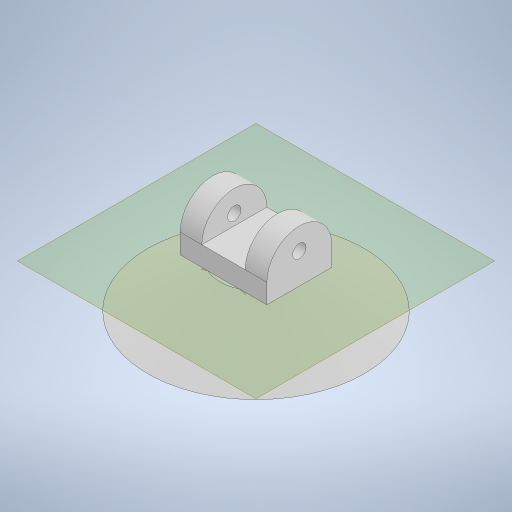
# Autodesk Inventor part: Деталь5
Saved by Autodesk Inventor 2023.1 (Build 271208000, 208)
## iProperties
Created: 2024-12-24
Part Number: Деталь5
Material: Типовые
Document SubType Name: Modeling
Designer: DELL
Density: 1 g/cm^3
Appearance: По умолчанию
Author: DELL
Autodesk Inventor part; units mm, degrees
ref_plane "YZ Plane" through (0, 0, 0) normal (1, 0, 0) x (0, 1, 0)
ref_plane "XZ Plane" through (0, 0, 0) normal (0, 1, 0) x (-1, 0, 0)
ref_plane "XY Plane" through (0, 0, 0) normal (0, 0, 1) x (1, 0, 0)
sketch "Эскиз2" plane through (0, 0, 0) normal (0, 0, 1) x (1, 0, 0)
  line L0 (0, 0) -> (25, 0)
  line L1 (0, 0) -> (0, 15)
  line L2 (0, 15) -> (25, 0)
  line L3 (0, -3) -> (0, 18) projected
  dimension "d0" = 25
  dimension "d1" = 15
  constraints: 6 end point, 1 horizontal, 1 vertical
  measures "d0" distance of L0.start L0.end
  measures "d1" distance of L0.start L1.end
revolve "Вращение1" add sketch "Эскиз2" angle 360 about axis through (0, -10, 0) along (0, 1, 0)
ref_plane "РабПлоскость1" through (0, 10, 0) normal (0, -1, 0) x (1, 0, 0)
sketch "Эскиз3" plane through (0, 10, 0) normal (0, -1, 0) x (1, 0, 0)
  line L0 (9.9198, 18.1472) -> (-9.6073, 18.1472)
  line L1 (-9.6073, 18.1472) -> (-9.6073, -14.8146)
  line L2 (-9.6073, -14.8146) -> (9.9198, -14.8146)
  line L3 (9.9198, -14.8146) -> (9.9198, 18.1472)
  point P0 (0, 0)
  constraints: 8 end point, 2 parallel, 1 horizontal, 1 perpendicular
extrude "Выдавливание1" cut sketch "Эскиз3" against normal blind 10
sketch "Эскиз4" plane through (0, 0, 0) normal (1, 0, 0) x (0, 1, 0)
  line L0 (14.521, 7.5) -> (0, 7.5)
  line L1 (0, 7.5) -> (0, -7.5)
  line L2 (0, -7.5) -> (14.521, -7.5)
  line L3 (14.521, -7.5) -> (14.521, 7.5)
  line L4 (14.521, 7.5) -> (0, -7.5) construction
  line L5 (0, 7.5) -> (14.521, -7.5) construction
  line L6 (10, 8.3333) -> (10, -8.3333) projected
  arc A0 (7.0249, 0.2433) -> (7.0249, -0.2433) centre (14.521, 0) ccw
  arc A1 (14.521, -7.5) -> (14.521, 7.5) centre (14.521, 0) ccw
  line L7 (14.521, 0) -> (17.021, 0) construction
  circle A2 centre (17.021, 0) radius 1.55
  point P0 (0, 0)
  point P1 (7.2605, 0)
  point P2 (10, 7.5)
  point P3 (10, -7.5)
  dimension "d6" = 15
  dimension "d7" = 4.521
  dimension "d10" = 2.5
  dimension "d11" = 3.1
  constraints: 14 end point, 4 point on circle, 3 centre point, 3 midpoint, 2 horizontal, 2 parallel, 2 point on line, 1 coincident, 1 perpendicular
  measures "d6" distance of L1.end L0.end
  measures "d7" distance from line of L2.end L6
  measures "d10" distance of L7.start L7.end
  measures "d11" diameter of A2
extrude "Выдавливание2" add sketch "Эскиз4" along normal mid plane 20 contours L3 L2 L6 L0 | A1 L3
extrude "Выдавливание3" cut sketch "Эскиз4" along normal mid plane 10 contours A1 L3 | L6 L2 L1 L0
